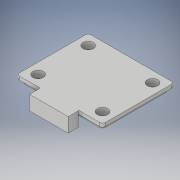
# Autodesk Inventor part: Enclosure_Top V4D6
Saved by Autodesk Inventor 2017 (Build 210142000, 142)
## iProperties
Created: 2017-12-18
Part Number: Enclosure_Top V4D6
Material: Generic
Document SubType Name: Modeling
Designer: Tripl_000
Density: 1 g/cm^3
Appearance: Default
Author: Tripl_000
Autodesk Inventor part; units mm, degrees
ref_plane "YZ Plane" through (0, 0, 0) normal (1, 0, 0) x (0, 1, 0)
ref_plane "XZ Plane" through (0, 0, 0) normal (0, 1, 0) x (-1, 0, 0)
ref_plane "XY Plane" through (0, 0, 0) normal (0, 0, 1) x (1, 0, 0)
sketch "Sketch1" plane through (0, 0, 0) normal (0, 1, 0) x (-1, 0, 0)
  line L0 (28, 23) -> (-28, 23)
  line L1 (-28, 23) -> (-28, -23)
  line L2 (-28, -23) -> (28, -23)
  line L3 (28, -23) -> (28, 23)
  line L4 (28, 23) -> (-28, -23) construction
  line L5 (-28, 23) -> (28, -23) construction
  point P0 (0, 0)
  dimension "d0" = 56
  dimension "d1" = 46
  constraints: 12 end point, 2 midpoint, 2 parallel, 1 horizontal, 1 perpendicular
  measures "d0" distance of L0.start L0.end
  measures "d1" distance of L2.end L0.start
extrude "Extrusion1" add sketch "Sketch1" along normal blind 2.5
sketch "Sketch2" plane through (0, 2.5, 0) normal (0, 1, 0) x (1, 0, 0)
  line L0 (-30, -25) -> (30, -25)
  line L1 (30, -25) -> (30, 25)
  line L2 (30, 25) -> (-30, 25)
  line L3 (-30, 25) -> (-30, -25)
  line L4 (-30, -25) -> (30, 25) construction
  line L5 (30, -25) -> (-30, 25) construction
  point P0 (0, 0)
  dimension "d4" = 50
  dimension "d5" = 60
  constraints: 12 end point, 2 midpoint, 2 parallel, 1 horizontal, 1 perpendicular
  measures "d4" distance of L2.end L0.start
  measures "d5" distance of L0.start L0.end
extrude "Extrusion2" add sketch "Sketch2" along normal blind 2.5
sketch "Sketch3" plane through (28, 0, 23) normal (1, 0, 0) x (0, 0, -1)
  line L0 (19.5, -2.5) -> (26.5, -2.5)
  line L1 (26.5, -2.5) -> (26.5, 2.5)
  line L2 (26.5, 2.5) -> (19.5, 2.5)
  line L3 (19.5, 2.5) -> (19.5, -2.5)
  line L4 (19.5, -2.5) -> (26.5, 2.5) construction
  line L5 (26.5, -2.5) -> (19.5, 2.5) construction
  point P0 (23, 0)
  dimension "d8" = 7
  dimension "d9" = 5
  constraints: 12 end point, 2 midpoint, 2 parallel, 1 horizontal, 1 perpendicular
  measures "d8" distance of L1.end L2.end
  measures "d9" distance of L0.end L1.end
extrude "Extrusion3" cut sketch "Sketch3" against normal through all
sketch "Sketch4" plane through (0, 5, 0) normal (0, 1, 0) x (1, 0, 0)
  line L0 (0, 31.16) -> (0, -35.6529)
  line L1 (-50.8705, 0) -> (45.6531, 0)
  circle A0 centre (-22.5, 17.5) radius 3.683
  circle A1 centre (22.5, 17.5) radius 3.683
  circle A2 centre (-22.5, -17.5) radius 3.683
  circle A3 centre (22.5, -17.5) radius 3.683
  point P0 (0, 0)
  dimension "d12" = 22.5
  dimension "d13" = 17.5
  dimension "d14" = 7.366
  constraints: 4 centre point, 4 end point, 3 symmetric about line, 1 horizontal, 1 vertical, 3 other
  measures "d12" horizontal distance of point (0, 0) A0.centre
  measures "d13" vertical distance of point (0, 0) A0.centre
  measures "d14" diameter of A0
fillet "Fillet1" radius 2 8 edges at (-28, 1.25, 23) (28, 1.25, 23) (28, 1.25, -23) (-28, 1.25, -23) (-30, 3.75, -25) (-30, 3.75, 25) (30, 3.75, 25) (30, 3.75, -25)
extrude "Extrusion5" cut sketch "Sketch4" against normal through all
sketch "Sketch5" plane through (-26, 0, 23) normal (0, 0, 1) x (1, 0, 0)
  line L0 (0, 2.5) -> (52, 2.5) projected
  line L1 (15, -2.5) -> (37, -2.5)
  line L2 (37, -2.5) -> (37, 2.5)
  line L3 (37, 2.5) -> (15, 2.5)
  line L4 (15, 2.5) -> (15, -2.5)
  line L5 (15, -2.5) -> (37, 2.5) construction
  line L6 (37, -2.5) -> (15, 2.5) construction
  point P0 (26, 0)
  dimension "d20" = 22
  constraints: 12 end point, 2 midpoint, 2 parallel, 1 horizontal, 1 perpendicular, 1 point on line
  measures "d20" distance of L1.start L1.end
extrude "Extrusion6" cut sketch "Sketch5" against normal through all
sketch "Sketch6" plane through (-28, 2.5, 25) normal (0, 0, 1) x (1, 0, 0)
  line L0 (17, 0) -> (17, -2.5) projected
  line L1 (56, 2.5) -> (0, 2.5) projected
  line L2 (17, 0) -> (39, 0)
  line L3 (39, 0) -> (39, 2.5)
  line L4 (39, 2.5) -> (17, 2.5)
  line L5 (17, 2.5) -> (17, 0)
  point P0 (28, -2.5)
  dimension "d23" = 22
  constraints: 8 end point, 2 parallel, 1 horizontal, 1 perpendicular, 1 point on line
  measures "d23" distance between parallel lines of L3 L5
extrude "Extrusion7" add sketch "Sketch6" along normal blind 10
sketch "Sketch7" plane through (0, 2.5, 0) normal (0, -1, 0) x (1, 0, 0)
  line L0 (-11, 25) -> (-11, 35) projected
  line L1 (11, 25) -> (11, 35) projected
  line L2 (-11, 35) -> (11, 35)
  line L3 (11, 35) -> (11, 30)
  line L4 (11, 30) -> (-11, 30)
  line L5 (-11, 30) -> (-11, 35)
  point P0 (0, 0)
  dimension "d26" = 5
  constraints: 8 end point, 2 parallel, 1 horizontal, 1 midpoint, 1 perpendicular
  measures "d26" distance between parallel lines of L4 L2
extrude "Extrusion8" add sketch "Sketch7" along normal blind 7.5
sketch "Sketch8" plane through (-11, 2.5, 25) normal (-1, 0, 0) x (0, 0, 1)
  line L0 (10, 2.5) -> (10, -7.5) projected
  line L1 (0, 2.5) -> (10, 2.5) projected
  line L2 (10, -7.5) -> (7.5, -7.5)
  line L3 (7.5, -7.5) -> (7.5, 2.5)
  line L4 (7.5, 2.5) -> (10, 2.5)
  line L5 (10, 2.5) -> (10, -7.5)
  point P0 (-25, -2.5)
  dimension "d29" = 2.5
  constraints: 8 end point, 2 parallel, 1 horizontal, 1 perpendicular, 1 point on line
  measures "d29" distance between parallel lines of L0 L3
extrude "Extrusion9" cut sketch "Sketch8" against normal through all
sketch "Sketch9" plane through (-11, -5, 32.5) normal (0, 0, 1) x (1, 0, 0)
  line L0 (0, 7.5) -> (0, 0) projected
  line L1 (39, 10) -> (-17, 10) projected
  line L2 (0, 0) -> (-2.5, 0)
  line L3 (-2.5, 0) -> (-2.5, 10)
  line L4 (-2.5, 10) -> (0, 10)
  line L5 (0, 10) -> (0, 0)
  line L6 (7.5, 20.7605) -> (7.5, -11.2566)
  line L7 (0, 0) -> (22, 0) projected
  line L8 (22, 0) -> (24.5, 0)
  line L9 (24.5, 0) -> (24.5, 10)
  line L10 (24.5, 10) -> (22, 10)
  line L11 (22, 10) -> (22, 0)
  point P0 (11, 5)
  dimension "d32" = 2.5
  dimension "d33" = 2.5
  constraints: 18 end point, 4 parallel, 2 horizontal, 2 perpendicular, 2 point on line, 1 vertical
  measures "d32" distance between parallel lines of L0 L3
  measures "d33" distance between parallel lines of L9 L11
extrude "Extrusion10" add sketch "Sketch9" against normal up to surface (7.5 mm away) contours L0 L2 L3 L1 L5 | L11 L1 L9 L8
ref_plane "Work Plane1" through (-28, 2.5, 0) normal (0, 0, 1) x (1, 0, 0)
mirror "Mirror1" about plane through (-28, 2.5, 0) normal (0, 0, 1) of "Extrusion7", "Extrusion8", "Extrusion9", "Extrusion10"
sketch "Sketch10" plane through (0, -5, 0) normal (0, -1, 0) x (1, 0, 0)
  line L0 (13.5, 25) -> (28, 25) projected
  line L1 (-13.5, 32.5) -> (-13.5, 25) projected
  line L2 (13.5, 25) -> (-13.5, 25)
  line L3 (-13.5, 25) -> (-13.5, 25.5)
  line L4 (-13.5, 25.5) -> (13.5, 25.5)
  line L5 (13.5, 25.5) -> (13.5, 25)
  line L6 (28, -25) -> (13.5, -25) projected
  line L7 (13.5, -25) -> (-13.5, -25)
  line L8 (-13.5, -25) -> (-13.5, -25.5)
  line L9 (-13.5, -25.5) -> (13.5, -25.5)
  line L10 (13.5, -25.5) -> (13.5, -25)
  point P0 (0, 0)
  dimension "d37" = 0.5
  dimension "d38" = 0.5
  constraints: 16 end point, 4 parallel, 2 horizontal, 2 perpendicular, 2 point on line
  measures "d37" distance between parallel lines of L4 L2
  measures "d38" distance between parallel lines of L7 L9
extrude "Extrusion11" cut sketch "Sketch10" against normal up to surface (7.5 mm away)
fillet "Fillet2" radius 5 2 edges at (0, 2.5, 30) (0, 2.5, -30)
ref_plane "Work Plane2" through (0, 2.5, 23) normal (1, 0, 0) x (0, 0, -1)
sketch "Sketch11" plane through (30, 2.5, 23) normal (1, 0, 0) x (0, 0, -1)
  line L0 (19.5, -2.5) -> (19.5, 0) projected
  line L1 (0, 2.5) -> (46, 2.5) projected
  line L2 (19.5, 0) -> (26.5, 0)
  line L3 (26.5, 0) -> (26.5, 2.5)
  line L4 (26.5, 2.5) -> (19.5, 2.5)
  line L5 (19.5, 2.5) -> (19.5, 0)
  point P0 (23, -2.5)
  dimension "d43" = 7
  constraints: 8 end point, 2 parallel, 1 horizontal, 1 perpendicular, 1 point on line
  measures "d43" distance between parallel lines of L3 L5
extrude "Extrusion12" add sketch "Sketch11" along normal blind 9.5
sketch "Sketch12" plane through (0, 2.5, 0) normal (0, -1, 0) x (1, 0, 0)
  line L0 (30, 3.5) -> (39.5, 3.5) projected
  line L1 (30, -3.5) -> (39.5, -3.5) projected
  line L2 (39.5, 3.5) -> (37, 3.5)
  line L3 (37, 3.5) -> (37, -3.5)
  line L4 (37, -3.5) -> (39.5, -3.5)
  line L5 (39.5, -3.5) -> (39.5, 3.5)
  point P0 (0, 0)
  dimension "d46" = 2.5
  constraints: 8 end point, 2 parallel, 1 horizontal, 1 perpendicular, 1 point on line
  measures "d46" distance between parallel lines of L3 L5
extrude "Extrusion13" add sketch "Sketch12" along normal blind 10
sketch "Sketch13" plane through (39.5, 2.5, 23) normal (1, 0, 0) x (0, 0, -1)
  line L0 (26.5, 2.5) -> (19.5, 2.5) projected
  line L1 (19.5, 2.5) -> (17, 2.5)
  line L2 (17, 2.5) -> (17, -10)
  line L3 (17, -10) -> (19.5, -10)
  line L4 (19.5, -10) -> (19.5, 2.5)
  line L5 (26.5, 2.5) -> (26.5, 0) projected
  line L6 (26.5, 2.5) -> (29, 2.5)
  line L7 (29, 2.5) -> (29, -10)
  line L8 (29, -10) -> (26.5, -10)
  line L9 (26.5, -10) -> (26.5, 2.5)
  point P0 (23, -2.5)
  dimension "d49" = 2.5
  dimension "d50" = 2.5
  constraints: 16 end point, 4 parallel, 2 horizontal, 2 perpendicular, 1 point on line
  measures "d49" distance between parallel lines of L4 L2
  measures "d50" distance between parallel lines of L9 L7
extrude "Extrusion14" add sketch "Sketch13" against normal up to surface (9.5 mm away)
sketch "Sketch14" plane through (0, -7.5, 0) normal (0, -1, 0) x (1, 0, 0)
  line L0 (30, 23) -> (30, 6) projected
  line L1 (39.5, -6) -> (30, -6) projected
  line L2 (30, 6) -> (30.5, 6)
  line L3 (30.5, 6) -> (30.5, -6)
  line L4 (30.5, -6) -> (30, -6)
  line L5 (30, -6) -> (30, 6)
  point P0 (0, 0)
  dimension "d53" = 0.5
  constraints: 8 end point, 2 parallel, 1 horizontal, 1 perpendicular, 1 point on line
  measures "d53" distance between parallel lines of L3 L5
extrude "Extrusion15" cut sketch "Sketch14" against normal up to surface (10 mm away)
mirror "Mirror2" about plane through (0, 2.5, 23) normal (1, 0, 0) of "Extrusion12", "Extrusion13", "Extrusion14", "Extrusion15"
fillet "Fillet3" radius 5 2 edges at (-37, 2.5, 0) (37, 2.5, 0)
sketch "Sketch15" plane through (39.5, -7.5, -6) normal (0, 0, -1) x (-1, 0, 0)
  line L0 (9.5, 12.5) -> (-10.1676, 12.5)
  line L1 (-10.1676, 12.5) -> (-10.1676, -21.7624)
  line L2 (-10.1676, -21.7624) -> (9.5, -21.7624)
  line L3 (9.5, -21.7624) -> (9.5, 12.5)
  point P0 (39.5, 7.5)
  constraints: 8 end point, 2 parallel, 1 horizontal, 1 perpendicular
extrude "Extrusion16" cut sketch "Sketch15" against normal through all
mirror "Mirror3" about plane through (0, 2.5, 23) normal (1, 0, 0) of "Extrusion16"
sketch "Sketch16" plane through (-13.5, -5, -32.5) normal (-1, 0, 0) x (0, 0, 1)
  line L0 (0, 10) -> (7.5, 10) projected
  line L1 (7.5, 10) -> (-5.2258, 10)
  line L2 (-5.2258, 10) -> (-5.2258, -4.6764)
  line L3 (-5.2258, -4.6764) -> (7.5, -4.6764)
  line L4 (7.5, -4.6764) -> (7.5, 10)
  point P0 (32.5, 5)
  constraints: 8 end point, 2 parallel, 1 horizontal, 1 perpendicular
extrude "Extrusion17" cut sketch "Sketch16" against normal through all
sketch "Sketch17" plane through (28, 0, -3.5) normal (0, 0, 1) x (1, 0, 0)
  line L0 (0, 0) -> (-17, 0) projected
  line L1 (0, 2.5) -> (-17, 2.5) projected
  line L2 (0, 0) -> (-1.5, 0)
  line L3 (-1.5, 0) -> (-1.5, 2.5)
  line L4 (-1.5, 2.5) -> (0, 2.5)
  line L5 (0, 2.5) -> (0, 0)
  line L6 (-56, 0) -> (-56, 2.5) projected
  line L7 (-39, 2.5) -> (-56, 2.5) projected
  line L8 (-56, 0) -> (-54.5, 0)
  line L9 (-54.5, 0) -> (-54.5, 2.5)
  line L10 (-54.5, 2.5) -> (-56, 2.5)
  line L11 (-56, 2.5) -> (-56, 0)
  point P0 (-28, 0)
  dimension "d69" = 1.5
  dimension "d70" = 1.5
  constraints: 16 end point, 4 parallel, 2 horizontal, 2 perpendicular, 2 point on line
  measures "d69" distance between parallel lines of L3 L5
  measures "d70" distance between parallel lines of L6 L9
extrude "Extrusion18" add sketch "Sketch17" along normal up to surface (7 mm away)
sketch "Sketch18" plane through (0, 2.5, 0) normal (0, -1, 0) x (1, 0, 0)
  line L0 (-11, -23) -> (11, -23)
  line L1 (11, -23) -> (11, -3.5)
  line L2 (11, -3.5) -> (-11, -3.5)
  line L3 (-11, -3.5) -> (-11, -23)
  point P0 (0, 0)
  constraints: 8 end point, 2 parallel, 1 horizontal, 1 perpendicular
extrude "Extrusion19" add sketch "Sketch18" along normal up to surface (2.5 mm away)
sketch "Sketch19" plane through (0, 2.5, 0) normal (0, -1, 0) x (1, 0, 0)
  line L0 (11, 23) -> (11, 3.5) projected
  line L1 (-11, 23) -> (-11, 3.5) projected
  line L2 (11, 10) -> (-11, 10)
  line L3 (-11, 10) -> (-11, 7.5)
  line L4 (-11, 7.5) -> (11, 7.5)
  line L5 (11, 7.5) -> (11, 10)
  line L6 (11, 23) -> (26, 23) projected
  point P0 (0, 0)
  dimension "d79" = 13
  dimension "d80" = 2.5
  constraints: 8 end point, 2 parallel, 2 point on line, 1 horizontal, 1 perpendicular
  measures "d79" distance between parallel lines of L6 L2
  measures "d80" distance between parallel lines of L4 L2
extrude "Extrusion20" cut sketch "Sketch19" against normal blind 1.5
sketch "Sketch20" plane through (0, 2.5, 0) normal (0, -1, 0) x (1, 0, 0)
  line L0 (11, 23) -> (11, 10) projected
  line L1 (-11, 3.5) -> (-11, 23) projected
  line L2 (11, 20.5) -> (-11, 20.5)
  line L3 (-11, 20.5) -> (-11, 3.5)
  line L4 (-11, 3.5) -> (11, 3.5)
  line L5 (11, 3.5) -> (11, 20.5)
  point P0 (0, 0)
  dimension "d83" = 17
  constraints: 8 end point, 2 parallel, 1 horizontal, 1 perpendicular, 1 point on line
  measures "d83" distance between parallel lines of L4 L2
extrude "Extrusion21" cut sketch "Sketch20" against normal up to surface (1.5 mm away)
sketch "Sketch21" plane through (0, 2.5, 0) normal (0, -1, 0) x (1, 0, 0)
  line L0 (-11, 3.5) -> (11, 3.5) projected
  line L1 (26.5, -3.5) -> (-26.5, -3.5) projected
  line L2 (11, 3.5) -> (-10.9417, 3.5)
  line L3 (-10.9417, 3.5) -> (-10.9417, -3.5)
  line L4 (-10.9417, -3.5) -> (11, -3.5)
  line L5 (11, -3.5) -> (11, 3.5)
  point P0 (0, 0)
  constraints: 8 end point, 2 parallel, 1 horizontal, 1 perpendicular, 1 point on line
extrude "Extrusion22" cut sketch "Sketch21" against normal up to surface (1.5 mm away)
sketch "Sketch22" plane through (0, 0, 0) normal (0, -1, 0) x (1, 0, 0)
  line L0 (26.5, -3.5) -> (26.5, 3.5) projected
  line L1 (26.5, -3.5) -> (-26.5, -3.5)
  line L2 (-26.5, -3.5) -> (-26.5, -10.5)
  line L3 (-26.5, -10.5) -> (26.5, -10.5)
  line L4 (26.5, -10.5) -> (26.5, -3.5)
  point P0 (0, 0)
  dimension "d88" = 7
  constraints: 8 end point, 2 parallel, 1 horizontal, 1 perpendicular
  measures "d88" distance between parallel lines of L3 L1
extrude "Extrusion23" cut sketch "Sketch22" against normal up to surface (2.5 mm away)
body "Solid1"
